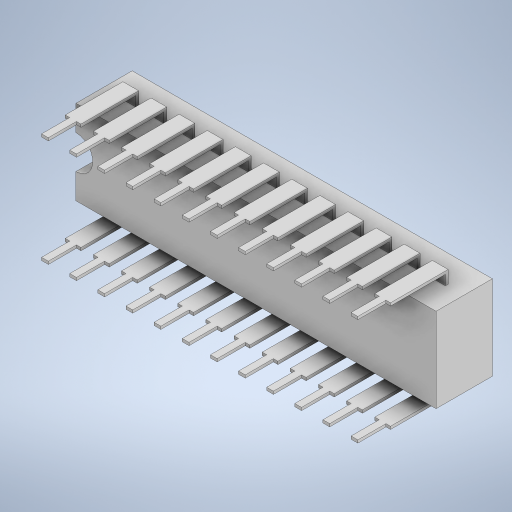
# Autodesk Inventor part: K555ID3
Saved by Autodesk Inventor 2023 (Build 270158000, 158)
## iProperties
Created: 2023-12-14
Part Number: K555ID3
Material: Generic
Document SubType Name: Sheet Metal
Designer: dank1
Density: 1 g/cm^3
Sheet Metal Rule: Default
Appearance: Default
Author: dank1
Autodesk Inventor part; units mm, degrees
ref_plane "YZ Plane" through (0, 0, 0) normal (1, 0, 0) x (0, 1, 0)
ref_plane "XZ Plane" through (0, 0, 0) normal (0, 1, 0) x (-1, 0, 0)
sketch "Sketch2" plane through (0, 0, 0) normal (0, 0, 1) x (1, 0, 0)
  line L0 (-16, 3.75) -> (16, 3.75)
  line L1 (16, 3.75) -> (16, -3.75)
  line L2 (16, -3.75) -> (-16, -3.75)
  line L3 (-16, -3.75) -> (-16, 3.75)
  line L4 (-16, 3.75) -> (16, -3.75) construction
  line L5 (16, 3.75) -> (-16, -3.75) construction
  point P0 (0, 0)
  dimension "d2" = 32
  dimension "d3" = 7.5
  constraints: 12 end point, 2 midpoint, 2 parallel, 1 horizontal, 1 perpendicular
  measures "d2" distance of L1.end L2.end
  measures "d3" distance of L0.end L1.end
extrude "Extrusion1" add sketch "Sketch2" along normal blind 5
ref_plane "Work Plane1" through (-13.75, -3.75, 0) normal (-1, 0, 0) x (0, 0, 1)
sketch "Sketch3" plane through (-13.75, -3.75, 0) normal (-1, 0, 0) x (0, 0, 1)
  line L0 (0, 7.5) -> (5, 7.5) projected
  line L1 (2.5, 7.5) -> (2.5, 8.5)
  line L2 (2.5, 7.5) -> (3.5, 7.5) construction
  line L3 (2.5, 8.5) -> (7.5, 8.5)
  point P0 (0, 3.75)
  dimension "d7" = 1
  dimension "d8" = 90
  dimension "d9" = 5
  constraints: 6 end point, 2 perpendicular, 1 horizontal, 1 midpoint, 1 vertical
  measures "d7" distance of L1.start L1.end
  measures "d8" angle of L2 L1
  measures "d9" distance of L1.end L3.end
sketch "Sketch4" plane through (-16, 3.75, 0) normal (0, 1, 0) x (1, 0, 0)
  line L0 (1.55, -2.375) -> (2.95, -2.375)
  line L1 (2.95, -2.375) -> (2.95, -2.625)
  line L2 (2.95, -2.625) -> (1.55, -2.625)
  line L3 (1.55, -2.625) -> (1.55, -2.375)
  line L4 (1.55, -2.375) -> (2.95, -2.625) construction
  line L5 (2.95, -2.375) -> (1.55, -2.625) construction
  point P0 (16, 0)
  point P1 (2.25, -2.5)
  dimension "d10" = 1.4
  dimension "d11" = 0.25
  constraints: 12 end point, 2 midpoint, 2 parallel, 1 horizontal, 1 perpendicular
  measures "d10" distance of L1.end L2.end
  measures "d11" distance of L0.end L1.end
sweep "Sweep1" add profiles "Sketch4" path "Sketch3" path curves L1 L3
sketch "Sketch5" plane through (-14.45, 4.625, 7.5) normal (0, 0, 1) x (1, 0, 0)
  line L0 (0, 0) -> (1.4, 0) projected
  line L1 (0.4, 0.25) -> (1, 0.25)
  line L2 (1, 0.25) -> (1, 0)
  line L3 (1, 0) -> (0.4, 0)
  line L4 (0.4, 0) -> (0.4, 0.25)
  line L5 (0.4, 0.25) -> (1, 0) construction
  line L6 (1, 0.25) -> (0.4, 0) construction
  point P0 (14.45, -4.625)
  point P1 (0.7, 0.125)
  point P2 (0.4, 0)
  dimension "d14" = 0.6
  constraints: 12 end point, 2 midpoint, 2 parallel, 1 horizontal, 1 perpendicular, 1 point on line
  measures "d14" distance of L2.end L3.end
extrude "Extrusion2" add sketch "Sketch5" along normal blind 2.5
pattern_linear "Rectangular Pattern1" count 12 spacing 2.5 along (1, 0, 0) of "Sweep1", "Extrusion2"
mirror "Mirror1" about plane through (0, 0, 0) normal (0, 1, 0) of "Sweep1", "Extrusion2", "Rectangular Pattern1"
sketch "Sketch6" plane through (0, 0, 0) normal (0, 0, -1) x (-1, 0, 0)
  line L0 (8.1679, -1.7458) -> (-9.1815, -1.7458) construction
  line L1 (-9.1815, -1.7458) -> (-9.1815, 2.0556) construction
  line L2 (-9.1815, 2.0556) -> (8.1679, 2.0556) construction
  line L3 (8.1679, 2.0556) -> (8.1679, -1.7458) construction
  point P0 (0, 0)
  constraints: 2 other
sketch "Sketch7" plane through (0, 0, 0) normal (0, 0, -1) x (-1, 0, 0)
  line L0 (16, 3.75) -> (16, -3.75) projected
  circle A0 centre (16, 0) radius 1.5
  point P0 (0, 0)
  dimension "d20" = 3
  constraints: 1 centre point, 1 midpoint
  measures "d20" diameter of A0
hole "Hole1" at (-16, 0, 0) direction (0, 0, 1) diameter 3 end through all
equation "\"d26\" = Thickness"
equation "\"BendRadius\" = Thickness"
equation "\"BendReliefWidth\" = Thickness"
equation "\"BendReliefDepth\" = 0.5 * Thickness"
equation "\"CornerReliefSize\" = 4 * Thickness"
equation "\"MinimumRemnant\" = 2 * Thickness"
equation "\"TransitionRadius\" = BendRadius"
equation "\"JacobiRadiusSize\" = BendRadius"
equation "\"GapSize\" = Thickness"
equation "\"Thickness\" = 3.048"
body "Solid1"
